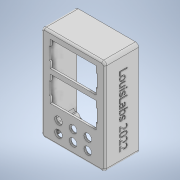
# Autodesk Inventor part: front_case
Saved by Autodesk Inventor 2022.1 (Build 261234020, 234B)
## iProperties
Created: 2022-02-06
Part Number: front_case
Material: Polylactic Acid (PLA)
Document SubType Name: Modeling
Designer: kee
Mass: 129.334 g
Surface Area: 618.34 cm^2
Volume: 103.468 cm^3
Density: 1.25 g/cm^3
Appearance: Default
Author: kee
Autodesk Inventor part; units mm, degrees
ref_plane "YZ Plane" through (0, 0, 0) normal (1, 0, 0) x (0, 1, 0)
ref_plane "XZ Plane" through (0, 0, 0) normal (0, 1, 0) x (-1, 0, 0)
ref_plane "XY Plane" through (0, 0, 0) normal (0, 0, 1) x (1, 0, 0)
sketch "Sketch1" plane through (0, 0, 0) normal (0, 0, 1) x (1, 0, 0)
  line L0 (-45, 75) -> (45, 75)
  line L1 (50, 70) -> (50, -70)
  line L2 (45, -75) -> (-45, -75)
  line L3 (-50, -70) -> (-50, 70)
  arc A0 (-45, 75) -> (-50, 70) centre (-45, 70) ccw
  arc A1 (50, 70) -> (45, 75) centre (45, 70) ccw
  arc A2 (-50, -70) -> (-45, -75) centre (-45, -70) ccw
  arc A3 (45, -75) -> (50, -70) centre (45, -70) ccw
  point P0 (0, 0)
  point P1 (-50, 75)
  point P2 (50, -75)
  point P3 (50, 75)
  point P4 (-50, -75)
  point P5 (50, 0)
  dimension "d3" = 100
  dimension "d4" = 50
  dimension "d5" = 150
  dimension "d6" = 75
  dimension "d37" = 5
  dimension "d125" = 90
  dimension "d126" = 140
  constraints: 8 end point, 8 point on circle, 8 point on line, 8 tangent, 4 centre point, 3 equal radius, 2 parallel, 1 horizontal, 1 midpoint, 1 perpendicular
  measures "d3" distance between parallel lines of L1 L3
  measures "d4" distance of point (50, 0) point (0, 0)
  measures "d5" distance between parallel lines of L2 L0
  measures "d6" distance from line of L2 point (0, 0)
  measures "d37" radius of A0
  measures "d125" distance of A0.centre A1.centre
  measures "d126" distance of A3.centre A1.centre
extrude "Extrusion1" add sketch "Sketch1" along normal blind 3
sketch "Sketch2" plane through (0, 0, 3) normal (0, 0, 1) x (1, 0, 0)
  circle A0 centre (-23, -40) radius 6
  circle A1 centre (-23, -58) radius 6
  circle A2 centre (0, -40) radius 6
  circle A3 centre (0, -58) radius 6
  circle A4 centre (23, -40) radius 6
  circle A5 centre (23, -58) radius 6
  line L0 (-45, -75) -> (45, -75) projected
  line L1 (-36, 17) -> (36, 17)
  line L2 (36, 17) -> (36, 7)
  line L3 (36, 7) -> (38, 7)
  line L4 (38, 7) -> (38, -13)
  line L5 (38, -13) -> (36, -13)
  line L6 (36, -13) -> (36, -23)
  line L7 (36, -23) -> (-36, -23)
  line L8 (-36, -23) -> (-36, -13)
  line L9 (-36, -13) -> (-38, -13)
  line L10 (-38, -13) -> (-38, 7)
  line L11 (-38, 7) -> (-36, 7)
  line L12 (-36, 17) -> (-36, 7)
  line L13 (-36, 64.5) -> (36, 64.5)
  line L14 (36, 64.5) -> (36, 54.5)
  line L15 (36, 54.5) -> (38, 54.5)
  line L16 (38, 54.5) -> (38, 34.5)
  line L17 (38, 34.5) -> (36, 34.5)
  line L18 (36, 34.5) -> (36, 24.5)
  line L19 (36, 24.5) -> (-36, 24.5)
  line L20 (-36, 24.5) -> (-36, 34.5)
  line L21 (-36, 34.5) -> (-38, 34.5)
  line L22 (-38, 34.5) -> (-38, 54.5)
  line L23 (-38, 54.5) -> (-36, 54.5)
  line L24 (-36, 64.5) -> (-36, 54.5)
  point P0 (-50, -70)
  point P1 (50, -70)
  point P2 (0, 0)
  point P3 (0, 47.5)
  dimension "d7" = 12
  dimension "d8" = 12
  dimension "d9" = 12
  dimension "d10" = 12
  dimension "d11" = 12
  dimension "d12" = 12
  dimension "d13" = 23
  dimension "d14" = 23
  dimension "d15" = 18
  dimension "d18" = 72
  dimension "d19" = 36
  dimension "d20" = 40
  dimension "d21" = 10
  dimension "d22" = 10
  dimension "d23" = 2
  dimension "d24" = 2
  dimension "d27" = 23
  dimension "d28" = 72
  dimension "d29" = 36
  dimension "d30" = 40
  dimension "d31" = 10
  dimension "d32" = 10
  dimension "d33" = 2
  dimension "d34" = 2
  dimension "d35" = 23
  dimension "d36" = 7.5
  dimension "d100" = 52
  dimension "d101" = 17
  constraints: 48 end point, 14 perpendicular, 14 point on line, 6 centre point, 4 horizontal alignment, 4 vertical alignment, 2 horizontal, 2 vertical, 1 other
  measures "d7" diameter of A0
  measures "d8" diameter of A1
  measures "d9" diameter of A2
  measures "d10" diameter of A3
  measures "d11" diameter of A4
  measures "d12" diameter of A5
  measures "d13" distance of A2.centre A0.centre
  measures "d14" distance of A4.centre A2.centre
  measures "d15" distance of A5.centre A4.centre
  measures "d18" distance of L1.start L1.end
  measures "d19" distance from line of L2 point (0, 0)
  measures "d20" distance between parallel lines of L7 L1
  measures "d21" distance of L1.end L2.end
  measures "d22" distance of L5.end L6.end
  measures "d23" distance between parallel lines of L4 L6
  measures "d24" distance between parallel lines of L10 L8
  measures "d27" distance from line of L7 point (0, 0)
  measures "d28" distance of L24.start L14.start
  measures "d29" distance from line of L14 point (0, 47.5)
  measures "d30" distance between parallel lines of L19 L13
  measures "d31" distance of L14.start L15.start
  measures "d32" distance of L18.start L19.start
  measures "d33" distance between parallel lines of L16 L18
  measures "d34" distance between parallel lines of L22 L20
  measures "d35" distance from line of L19 point (0, 47.5)
  measures "d36" distance between parallel lines of L1 L19
  measures "d100" vertical distance of point (45, -75) L6.end
  measures "d101" distance from line of L7 A4.centre
extrude "Extrusion2" cut sketch "Sketch2" against normal up to next
sketch "Sketch5" plane through (0, 0, 0) normal (0, 0, -1) x (-1, 0, 0)
  circle A0 centre (23, -40) radius 6 projected
  circle A1 centre (0, -58) radius 6 projected
  circle A2 centre (23, -58) radius 6 projected
  line L0 (38, 7) -> (38, -13) projected
  line L1 (38, -13) -> (36, -13) projected
  line L2 (36, -13) -> (36, -23) projected
  line L3 (36, -23) -> (-36, -23) projected
  line L4 (-36, -23) -> (-36, -13) projected
  line L5 (-36, -13) -> (-38, -13) projected
  line L6 (-38, -13) -> (-38, 7) projected
  line L7 (-38, 7) -> (-36, 7) projected
  line L8 (-36, 7) -> (-36, 17) projected
  line L9 (-36, 17) -> (36, 17) projected
  line L10 (36, 17) -> (36, 7) projected
  line L11 (36, 7) -> (38, 7) projected
  circle A3 centre (0, -40) radius 6 projected
  circle A4 centre (-23, -58) radius 6 projected
  circle A5 centre (-23, -40) radius 6 projected
  line L12 (38, 54.5) -> (38, 34.5) projected
  line L13 (38, 34.5) -> (36, 34.5) projected
  line L14 (36, 34.5) -> (36, 24.5) projected
  line L15 (36, 24.5) -> (-36, 24.5) projected
  line L16 (-36, 24.5) -> (-36, 34.5) projected
  line L17 (-36, 34.5) -> (-38, 34.5) projected
  line L18 (-38, 34.5) -> (-38, 54.5) projected
  line L19 (-38, 54.5) -> (-36, 54.5) projected
  line L20 (-36, 54.5) -> (-36, 64.5) projected
  line L21 (-36, 64.5) -> (36, 64.5) projected
  line L22 (36, 64.5) -> (36, 54.5) projected
  line L23 (36, 54.5) -> (38, 54.5) projected
  line L24 (45, -75) -> (-45, -75) projected
  arc A6 (45, -75) -> (50, -70) centre (45, -70) ccw projected
  line L25 (50, 70) -> (50, -70) projected
  arc A7 (50, 70) -> (45, 75) centre (45, 70) ccw projected
  line L26 (-45, 75) -> (45, 75) projected
  arc A8 (-45, 75) -> (-50, 70) centre (-45, 70) ccw projected
  line L27 (-50, -70) -> (-50, 70) projected
  arc A9 (-50, -70) -> (-45, -75) centre (-45, -70) ccw projected
  arc A10 (47, 70) -> (45, 72) centre (45, 70) ccw
  line L28 (47, 70) -> (47, -70)
  arc A11 (45, -72) -> (47, -70) centre (45, -70) ccw
  line L29 (45, -72) -> (-45, -72)
  arc A12 (-47, -70) -> (-45, -72) centre (-45, -70) ccw
  line L30 (-47, -70) -> (-47, 70)
  arc A13 (-45, 72) -> (-47, 70) centre (-45, 70) ccw
  line L31 (-45, 72) -> (45, 72)
  line L32 (-45, 75) -> (45, 75)
  arc A14 (50, 70) -> (45, 75) centre (45, 70) ccw
  line L33 (50, 70) -> (50, -70)
  arc A15 (45, -75) -> (50, -70) centre (45, -70) ccw
  line L34 (45, -75) -> (-45, -75)
  arc A16 (-50, -70) -> (-45, -75) centre (-45, -70) ccw
  line L35 (-50, -70) -> (-50, 70)
  arc A17 (-45, 75) -> (-50, 70) centre (-45, 70) ccw
  line L36 (-116.3396, 0) -> (109.1655, 0) construction
  line L37 (0, 86.6309) -> (0, -88.1774) construction
  line L38 (-47, 62) -> (-42, 62)
  line L39 (-37, 67) -> (-37, 72)
  arc A18 (-42, 62) -> (-37, 67) centre (-42, 67) ccw
  line L40 (47, 62) -> (42, 62)
  line L41 (37, 67) -> (37, 72)
  arc A19 (37, 67) -> (42, 62) centre (42, 67) ccw
  line L42 (37, -72) -> (37, -67)
  line L43 (42, -62) -> (47, -62)
  arc A20 (42, -62) -> (37, -67) centre (42, -67) ccw
  line L44 (-37, -72) -> (-37, -67)
  line L45 (-42, -62) -> (-47, -62)
  arc A21 (-37, -67) -> (-42, -62) centre (-42, -67) ccw
  point P0 (0, 0)
  point P1 (-37, 62)
  point P2 (37, 62)
  point P3 (37, -62)
  point P4 (-37, -62)
  dimension "d38" = 3
  dimension "d103" = 10
  dimension "d104" = 10
  dimension "d105" = 5
  dimension "d108" = 10
  dimension "d109" = 10
  dimension "d110" = 5
  dimension "d111" = 10
  dimension "d112" = 10
  dimension "d113" = 5
  dimension "d114" = 10
  dimension "d115" = 10
  dimension "d116" = 5
  dimension "d127" = 84
  dimension "d128" = 134
  constraints: 36 end point, 24 point on circle, 18 point on line, 13 tangent, 12 centre point, 5 perpendicular, 4 coincident, 4 horizontal, 4 vertical, 7 other
  measures "d38" distance between parallel lines of L26 L31
  measures "d103" distance of L38.start point (-37, 62)
  measures "d104" distance of point (-37, 62) L39.end
  measures "d105" radius of A18
  measures "d108" distance of L40.start point (37, 62)
  measures "d109" distance of point (37, 62) L41.end
  measures "d110" radius of A19
  measures "d111" distance of L42.start point (37, -62)
  measures "d112" distance of point (37, -62) L43.end
  measures "d113" radius of A20
  measures "d114" distance of L44.start point (-37, -62)
  measures "d115" distance of point (-37, -62) L45.end
  measures "d116" radius of A21
  measures "d127" distance of A19.centre A18.centre
  measures "d128" distance of A20.centre A19.centre
extrude "Extrusion13" add sketch "Sketch5" along normal blind 50 contours L24 A9 L27 A8 L26 A7 L25 A6 | L28 L40 A19 L41 L31 A10 | L28 A11 L29 L42 A20 L43 | L39 A18 L38 L30 A13 L31 | L29 A12 L30 L45 A21 L44
sketch "Sketch17" plane through (0, 0, -50) normal (0, 0, -1) x (-1, 0, 0)
  line L0 (-45, -75) -> (45, -75) projected
  arc A0 (45, -75) -> (50, -70) centre (45, -70) ccw projected
  line L1 (50, -70) -> (50, 70) projected
  arc A1 (50, 70) -> (45, 75) centre (45, 70) ccw projected
  line L2 (45, 75) -> (-45, 75) projected
  arc A2 (-45, 75) -> (-50, 70) centre (-45, 70) ccw projected
  line L3 (-50, 70) -> (-50, -70) projected
  arc A3 (-50, -70) -> (-45, -75) centre (-45, -70) ccw projected
  line L4 (37, 72) -> (37, 67) projected
  arc A4 (37, 67) -> (42, 62) centre (42, 67) ccw projected
  line L5 (42, 62) -> (47, 62) projected
  line L6 (47, 62) -> (47, -62) projected
  line L7 (47, -62) -> (42, -62) projected
  arc A5 (42, -62) -> (37, -67) centre (42, -67) ccw projected
  line L8 (37, -67) -> (37, -72) projected
  line L9 (37, -72) -> (-37, -72) projected
  line L10 (-37, -72) -> (-37, -67) projected
  arc A6 (-37, -67) -> (-42, -62) centre (-42, -67) ccw projected
  line L11 (-42, -62) -> (-47, -62) projected
  line L12 (-47, -62) -> (-47, 62) projected
  line L13 (-47, 62) -> (-42, 62) projected
  arc A7 (-42, 62) -> (-37, 67) centre (-42, 67) ccw projected
  line L14 (-37, 67) -> (-37, 72) projected
  line L15 (-37, 72) -> (37, 72) projected
  line L16 (-42, 72) -> (42, 72)
  line L17 (47, 67) -> (47, -67)
  line L18 (42, -72) -> (-42, -72)
  line L19 (-47, -67) -> (-47, 67)
  arc A8 (-42, 72) -> (-47, 67) centre (-42, 67) ccw
  arc A9 (47, 67) -> (42, 72) centre (42, 67) ccw
  arc A10 (42, -72) -> (47, -67) centre (42, -67) ccw
  arc A11 (-47, -67) -> (-42, -72) centre (-42, -67) ccw
  point P0 (0, 0)
  point P1 (-47, 72)
  point P2 (-47, 62)
  dimension "d117" = 5
  constraints: 8 end point, 8 point on circle, 8 tangent, 4 centre point, 3 equal radius, 3 point on line, 2 parallel, 1 horizontal, 1 perpendicular
  measures "d117" radius of A8
extrude "Extrusion14" cut sketch "Sketch17" against normal blind 5 contours L16 A9 L17 L5 A4 L4 | L4 A4 L5 L6 L7 A5 L8 L9 L10 A6 L11 L12 L13 A7 L14 L15 | L14 A7 L13 L19 A8 L16 | L17 A10 L18 L8 A5 L7 | L11 A6 L10 L18 A11 L19
sketch "Sketch18" plane through (-45, -75, 3) normal (0, -1, 0) x (1, 0, 0)
  line L0 (3, -53) -> (87, -53) projected
  line L1 (85, -53) -> (5, -53)
  line L2 (5, -53) -> (5, -10)
  line L3 (5, -10) -> (85, -10)
  line L4 (85, -10) -> (85, -53)
  line L5 (0, 0) -> (90, 0) projected
  line L6 (45, -65.8831) -> (45, 5.9535) construction
  point P0 (45, -3)
  point P1 (45, 0)
  point P2 (5, -53)
  dimension "d120" = 10
  dimension "d121" = 80
  dimension "d122" = 40
  constraints: 10 end point, 2 parallel, 2 point on line, 1 horizontal, 1 midpoint, 1 perpendicular, 1 vertical
  measures "d120" distance between parallel lines of L5 L3
  measures "d121" distance between parallel lines of L2 L4
  measures "d122" distance between parallel lines of L2 L6
extrude "Extrusion15" cut sketch "Sketch18" against normal up to surface (3 mm away)
fillet "Fillet1" radius 3 2 edges at (40, -73.5, -7) (-40, -73.5, -7)
sketch "Sketch19" plane through (0, 0, -45) normal (0, 0, -1) x (-1, 0, 0)
  line L0 (-42, 62) -> (-47, 62) construction
  arc A0 (-42, 62) -> (-37, 67) centre (-42, 67) ccw construction
  line L1 (-37, 72) -> (-37, 67) construction
  line L2 (-42, 72) -> (-37, 72) construction
  arc A1 (-42, 72) -> (-47, 67) centre (-42, 67) ccw construction
  line L3 (-47, 62) -> (-47, 67) construction
  line L4 (47, 62) -> (42, 62) construction
  line L5 (47, 67) -> (47, 62) construction
  arc A2 (47, 67) -> (42, 72) centre (42, 67) ccw construction
  line L6 (37, 72) -> (42, 72) construction
  line L7 (37, 67) -> (37, 72) construction
  arc A3 (37, 67) -> (42, 62) centre (42, 67) ccw construction
  line L8 (37, -72) -> (37, -67) construction
  line L9 (40, -72) -> (37, -72) construction
  line L10 (42, -72) -> (40, -72) construction
  arc A4 (42, -72) -> (47, -67) centre (42, -67) ccw construction
  line L11 (47, -62) -> (47, -67) construction
  line L12 (42, -62) -> (47, -62) construction
  arc A5 (42, -62) -> (37, -67) centre (42, -67) ccw construction
  line L13 (-37, -67) -> (-37, -72) construction
  arc A6 (-37, -67) -> (-42, -62) centre (-42, -67) ccw construction
  line L14 (-47, -62) -> (-42, -62) construction
  line L15 (-47, -67) -> (-47, -62) construction
  arc A7 (-47, -67) -> (-42, -72) centre (-42, -67) ccw construction
  line L16 (-40, -72) -> (-42, -72) construction
  line L17 (-37, -72) -> (-40, -72) construction
  point P0 (0, 0)
hole "Hole1" at (42, 67, -45) at (-42, 67, -45) at (-42, -67, -45) at (42, -67, -45) direction (0, 0, 1) diameter 3 depth 15 tip angle 118
fillet "Fillet2" radius 3 29 edges at (48.5355, 73.5355, 3) (0, 75, 3) (-48.5355, 73.5355, 3) (-50, 0, 3) (-48.5355, -73.5355, 3) (0, -75, 3) (48.5355, -73.5355, 3) (50, 0, 3) (47, 62, -22.5) (37, 72, -22.5) (-47, 62, -22.5) (-37, 72, -22.5) (-47, -62, -22.5) (47, -62, -22.5) (47, 0, 0) (37, -69.5, 0) (44.5, -62, 0) (38.4645, -63.4645, 0) (-38.4645, -63.4645, 0) (-44.5, -62, 0) (-37, -69.5, 0) (0, -72, 0) (0, 72, 0) (38.4645, 63.4645, 0) (44.5, 62, 0) (37, 69.5, 0) (-38.4645, 63.4645, 0) (-44.5, 62, 0) (-37, 69.5, 0)
sketch "Sketch20" plane through (50, -70, -50) normal (1, 0, 0) x (0, 0, -1)
  line L0 (-30.2308, 115.0433) -> (-30.2308, 121.9963)
  line L1 (-30.2308, 121.9963) -> (-18.2308, 121.9963)
  line L2 (-18.2308, 121.9963) -> (-18.2308, 120.4015)
  line L3 (-18.2308, 120.4015) -> (-28.811, 120.4015)
  line L4 (-28.811, 120.4015) -> (-28.811, 115.0433)
  line L5 (-28.811, 115.0433) -> (-30.2308, 115.0433)
  spline S0 degree 2 poles (-25.7284, 106.5052) (-28.0039, 106.5052) (-30.4836, 108.6932) (-30.4836, 110.5214) knots 0 0 0 1 2 2 2
  spline S1 degree 2 poles (-30.4836, 110.5214) (-30.4836, 112.3982) (-27.9261, 114.5474) (-25.7284, 114.5474) knots 0 0 0 1 2 2 2
  spline S2 degree 2 poles (-25.7284, 114.5474) (-23.4723, 114.5474) (-20.9731, 112.3302) (-20.9731, 110.5214) knots 0 0 0 1 2 2 2
  spline S3 degree 2 poles (-20.9731, 110.5214) (-20.9731, 108.6932) (-23.4626, 106.5052) (-25.7284, 106.5052) knots 0 0 0 1 2 2 2
  spline S4 degree 2 poles (-25.7284, 108.0709) (-23.9779, 108.0709) (-22.2762, 109.3448) (-22.2762, 110.5214) knots 0 0 0 1 2 2 2
  spline S5 degree 2 poles (-22.2762, 110.5214) (-22.2762, 111.6981) (-23.9779, 112.9817) (-25.7284, 112.9817) knots 0 0 0 1 2 2 2
  spline S6 degree 2 poles (-25.7284, 112.9817) (-27.4301, 112.9817) (-29.1805, 111.6981) (-29.1805, 110.5214) knots 0 0 0 1 2 2 2
  spline S7 degree 2 poles (-29.1805, 110.5214) (-29.1805, 109.3545) (-27.4593, 108.0709) (-25.7284, 108.0709) knots 0 0 0 1 2 2 2
  line L6 (-30.2308, 97.9477) -> (-30.2308, 99.4647)
  line L7 (-30.2308, 99.4647) -> (-29.2389, 99.4647)
  spline S8 degree 2 poles (-29.2389, 99.4647) (-29.8515, 100.1649) (-30.4836, 101.4193) (-30.4836, 102.1973) knots 0 0 0 1 2 2 2
  spline S9 degree 2 poles (-30.4836, 102.1973) (-30.4836, 102.7807) (-30.0946, 103.8213) (-29.6765, 104.2005) knots 0 0 0 1 2 2 2
  spline S10 degree 2 poles (-29.6765, 104.2005) (-29.2583, 104.5895) (-27.9844, 105.0174) (-27.0703, 105.0174) knots 0 0 0 1 2 2 2
  line L8 (-27.0703, 105.0174) -> (-21.2259, 105.0174)
  line L9 (-21.2259, 105.0174) -> (-21.2259, 103.5004)
  line L10 (-21.2259, 103.5004) -> (-26.3604, 103.5004)
  spline S11 degree 2 poles (-26.3604, 103.5004) (-27.0801, 103.5004) (-28.0233, 103.3934) (-28.3734, 103.2086) knots 0 0 0 1 2 2 2
  spline S12 degree 2 poles (-28.3734, 103.2086) (-28.7235, 103.0239) (-29.0444, 102.3918) (-29.0444, 101.7986) knots 0 0 0 1 2 2 2
  spline S13 degree 2 poles (-29.0444, 101.7986) (-29.0444, 101.2443) (-28.4123, 99.9898) (-27.9553, 99.4647) knots 0 0 0 1 2 2 2
  line L11 (-27.9553, 99.4647) -> (-21.2259, 99.4647)
  line L12 (-21.2259, 99.4647) -> (-21.2259, 97.9477)
  line L13 (-21.2259, 97.9477) -> (-30.2308, 97.9477)
  line L14 (-30.2308, 94.2038) -> (-30.2308, 95.7208)
  line L15 (-30.2308, 95.7208) -> (-21.2259, 95.7208)
  line L16 (-21.2259, 95.7208) -> (-21.2259, 94.2038)
  line L17 (-21.2259, 94.2038) -> (-30.2308, 94.2038)
  line L18 (-19.7284, 94.0968) -> (-19.7284, 95.818)
  line L19 (-19.7284, 95.818) -> (-18.153, 95.818)
  line L20 (-18.153, 95.818) -> (-18.153, 94.0968)
  line L21 (-18.153, 94.0968) -> (-19.7284, 94.0968)
  spline S14 degree 2 poles (-30.4447, 89.5457) (-30.4447, 90.4501) (-29.9585, 92.0158) (-29.6862, 92.5311) knots 0 0 0 1 2 2 2
  line L22 (-29.6862, 92.5311) -> (-27.9844, 92.5311)
  line L23 (-27.9844, 92.5311) -> (-27.9844, 92.4534)
  spline S15 degree 2 poles (-27.9844, 92.4534) (-28.14, 92.2589) (-28.5096, 91.7337) (-28.7138, 91.2961) knots 0 0 0 1 2 2 2
  spline S16 degree 2 poles (-28.7138, 91.2961) (-28.8985, 90.9169) (-29.1708, 89.9833) (-29.1708, 89.4874) knots 0 0 0 1 2 2 2
  spline S17 degree 2 poles (-29.1708, 89.4874) (-29.1708, 89.1276) (-29.0055, 88.301) (-28.8694, 88.1065) knots 0 0 0 1 2 2 2
  spline S18 degree 2 poles (-28.8694, 88.1065) (-28.6846, 87.8245) (-28.2664, 87.5717) (-27.8386, 87.5717) knots 0 0 0 1 2 2 2
  spline S19 degree 2 poles (-27.8386, 87.5717) (-27.3037, 87.5717) (-26.7494, 88.1551) (-26.5647, 88.9039) knots 0 0 0 1 2 2 2
  spline S20 degree 2 poles (-26.5647, 88.9039) (-26.4966, 89.1957) (-26.3021, 90.1292) (-26.1951, 90.5279) knots 0 0 0 1 2 2 2
  spline S21 degree 2 poles (-26.1951, 90.5279) (-25.8937, 91.5587) (-24.6489, 92.4923) (-23.764, 92.4923) knots 0 0 0 1 2 2 2
  spline S22 degree 2 poles (-23.764, 92.4923) (-22.5387, 92.4923) (-21.012, 90.6543) (-21.012, 89.1373) knots 0 0 0 1 2 2 2
  spline S23 degree 2 poles (-21.012, 89.1373) (-21.012, 88.3885) (-21.3815, 86.8715) (-21.6635, 86.3561) knots 0 0 0 1 2 2 2
  line L24 (-21.6635, 86.3561) -> (-23.2875, 86.3561)
  line L25 (-23.2875, 86.3561) -> (-23.2875, 86.4339)
  spline S24 degree 2 poles (-23.2875, 86.4339) (-22.8207, 87.0174) (-22.2859, 88.4371) (-22.2859, 89.1665) knots 0 0 0 1 2 2 2
  spline S25 degree 2 poles (-22.2859, 89.1665) (-22.2859, 89.9153) (-22.918, 90.9461) (-23.5501, 90.9461) knots 0 0 0 1 2 2 2
  spline S26 degree 2 poles (-23.5501, 90.9461) (-24.1238, 90.9461) (-24.6781, 90.3334) (-24.8532, 89.6527) knots 0 0 0 1 2 2 2
  spline S27 degree 2 poles (-24.8532, 89.6527) (-24.9407, 89.3221) (-25.1157, 88.4858) (-25.2227, 88.0287) knots 0 0 0 1 2 2 2
  spline S28 degree 2 poles (-25.2227, 88.0287) (-25.4755, 87.0368) (-26.6327, 86.0255) (-27.6343, 86.0255) knots 0 0 0 1 2 2 2
  spline S29 degree 2 poles (-27.6343, 86.0255) (-28.2178, 86.0255) (-29.2486, 86.4825) (-29.6279, 86.9299) knots 0 0 0 1 2 2 2
  spline S30 degree 2 poles (-29.6279, 86.9299) (-30.0266, 87.4064) (-30.4447, 88.6219) (-30.4447, 89.5457) knots 0 0 0 1 2 2 2
  line L26 (-30.2308, 77.5457) -> (-30.2308, 84.4987)
  line L27 (-30.2308, 84.4987) -> (-18.2308, 84.4987)
  line L28 (-18.2308, 84.4987) -> (-18.2308, 82.9039)
  line L29 (-18.2308, 82.9039) -> (-28.811, 82.9039)
  line L30 (-28.811, 82.9039) -> (-28.811, 77.5457)
  line L31 (-28.811, 77.5457) -> (-30.2308, 77.5457)
  spline S31 degree 2 poles (-29.2778, 71.3901) (-29.4139, 71.5749) (-29.9002, 72.1973) (-30.046, 72.489) knots 0 0 0 1 2 2 2
  spline S32 degree 2 poles (-30.046, 72.489) (-30.26, 72.8877) (-30.4836, 73.6365) (-30.4836, 74.3172) knots 0 0 0 1 2 2 2
  spline S33 degree 2 poles (-30.4836, 74.3172) (-30.4836, 74.8715) (-30.0655, 75.8731) (-29.6862, 76.2524) knots 0 0 0 1 2 2 2
  spline S34 degree 2 poles (-29.6862, 76.2524) (-29.3167, 76.6122) (-28.2275, 77.0498) (-27.6246, 77.0498) knots 0 0 0 1 2 2 2
  spline S35 degree 2 poles (-27.6246, 77.0498) (-26.6911, 77.0498) (-25.3685, 76.2621) (-24.9893, 75.4064) knots 0 0 0 1 2 2 2
  spline S36 degree 2 poles (-24.9893, 75.4064) (-24.6392, 74.6478) (-24.3767, 72.5863) (-24.3086, 71.3901) knots 0 0 0 1 2 2 2
  line L32 (-24.3086, 71.3901) -> (-24.0168, 71.3901)
  spline S37 degree 2 poles (-24.0168, 71.3901) (-23.4917, 71.3901) (-22.8402, 71.7111) (-22.6554, 72.0028) knots 0 0 0 1 2 2 2
  spline S38 degree 2 poles (-22.6554, 72.0028) (-22.4707, 72.2945) (-22.354, 73.1308) (-22.354, 73.5782) knots 0 0 0 1 2 2 2
  spline S39 degree 2 poles (-22.354, 73.5782) (-22.354, 74.1033) (-22.6651, 75.523) (-22.9666, 76.2329) knots 0 0 0 1 2 2 2
  line L33 (-22.9666, 76.2329) -> (-22.9666, 76.3205)
  line L34 (-22.9666, 76.3205) -> (-21.4204, 76.3205)
  spline S40 degree 2 poles (-21.4204, 76.3205) (-21.3037, 75.9023) (-21.012, 74.3367) (-21.012, 73.5684) knots 0 0 0 1 2 2 2
  spline S41 degree 2 poles (-21.012, 73.5684) (-21.012, 72.6349) (-21.3037, 71.361) (-21.683, 70.8553) knots 0 0 0 1 2 2 2
  spline S42 degree 2 poles (-21.683, 70.8553) (-22.0525, 70.3593) (-23.2292, 69.8731) (-24.0752, 69.8731) knots 0 0 0 1 2 2 2
  line L35 (-24.0752, 69.8731) -> (-30.2308, 69.8731)
  line L36 (-30.2308, 69.8731) -> (-30.2308, 71.3901)
  line L37 (-30.2308, 71.3901) -> (-29.2778, 71.3901)
  line L38 (-28.0136, 71.3901) -> (-25.5144, 71.3901)
  spline S43 degree 2 poles (-25.5144, 71.3901) (-25.563, 71.9347) (-25.7284, 73.5782) (-25.8839, 74.0935) knots 0 0 0 1 2 2 2
  spline S44 degree 2 poles (-25.8839, 74.0935) (-26.0687, 74.6965) (-26.8369, 75.4841) (-27.5177, 75.4841) knots 0 0 0 1 2 2 2
  spline S45 degree 2 poles (-27.5177, 75.4841) (-28.2956, 75.4841) (-29.0833, 74.6089) (-29.0833, 73.7726) knots 0 0 0 1 2 2 2
  spline S46 degree 2 poles (-29.0833, 73.7726) (-29.0833, 73.0628) (-28.4707, 71.8958) (-28.0136, 71.3901) knots 0 0 0 1 2 2 2
  spline S47 degree 2 poles (-25.5825, 60.1973) (-27.7899, 60.1973) (-30.4836, 62.3367) (-30.4836, 63.9509) knots 0 0 0 1 2 2 2
  spline S48 degree 2 poles (-30.4836, 63.9509) (-30.4836, 64.6803) (-30.1238, 65.7208) (-29.8126, 66.2264) knots 0 0 0 1 2 2 2
  line L39 (-29.8126, 66.2264) -> (-30.2308, 66.3237)
  line L40 (-30.2308, 66.3237) -> (-30.2308, 67.7435)
  line L41 (-30.2308, 67.7435) -> (-17.6959, 67.7435)
  line L42 (-17.6959, 67.7435) -> (-17.6959, 66.2264)
  line L43 (-17.6959, 66.2264) -> (-22.1692, 66.2264)
  spline S49 degree 2 poles (-22.1692, 66.2264) (-21.6538, 65.6527) (-20.9731, 64.3205) (-20.9731, 63.4744) knots 0 0 0 1 2 2 2
  spline S50 degree 2 poles (-20.9731, 63.4744) (-20.9731, 61.9477) (-23.4139, 60.1973) (-25.5825, 60.1973) knots 0 0 0 1 2 2 2
  spline S51 degree 2 poles (-25.6992, 61.7629) (-24.0849, 61.7629) (-22.4123, 62.7451) (-22.4123, 63.8342) knots 0 0 0 1 2 2 2
  spline S52 degree 2 poles (-22.4123, 63.8342) (-22.4123, 64.4469) (-22.9958, 65.7111) (-23.4431, 66.2264) knots 0 0 0 1 2 2 2
  line L44 (-23.4431, 66.2264) -> (-28.6068, 66.2264)
  spline S53 degree 2 poles (-28.6068, 66.2264) (-28.8888, 65.6527) (-29.1222, 64.7678) (-29.1222, 64.2427) knots 0 0 0 1 2 2 2
  spline S54 degree 2 poles (-29.1222, 64.2427) (-29.1222, 63.0854) (-27.4788, 61.7629) (-25.6992, 61.7629) knots 0 0 0 1 2 2 2
  spline S55 degree 2 poles (-30.4447, 56.1908) (-30.4447, 57.0952) (-29.9585, 58.6608) (-29.6862, 59.1762) knots 0 0 0 1 2 2 2
  line L45 (-29.6862, 59.1762) -> (-27.9844, 59.1762)
  line L46 (-27.9844, 59.1762) -> (-27.9844, 59.0984)
  spline S56 degree 2 poles (-27.9844, 59.0984) (-28.14, 58.9039) (-28.5096, 58.3788) (-28.7138, 57.9412) knots 0 0 0 1 2 2 2
  spline S57 degree 2 poles (-28.7138, 57.9412) (-28.8985, 57.5619) (-29.1708, 56.6284) (-29.1708, 56.1324) knots 0 0 0 1 2 2 2
  spline S58 degree 2 poles (-29.1708, 56.1324) (-29.1708, 55.7726) (-29.0055, 54.9461) (-28.8694, 54.7516) knots 0 0 0 1 2 2 2
  spline S59 degree 2 poles (-28.8694, 54.7516) (-28.6846, 54.4696) (-28.2664, 54.2167) (-27.8386, 54.2167) knots 0 0 0 1 2 2 2
  spline S60 degree 2 poles (-27.8386, 54.2167) (-27.3037, 54.2167) (-26.7494, 54.8002) (-26.5647, 55.549) knots 0 0 0 1 2 2 2
  spline S61 degree 2 poles (-26.5647, 55.549) (-26.4966, 55.8407) (-26.3021, 56.7743) (-26.1951, 57.173) knots 0 0 0 1 2 2 2
  spline S62 degree 2 poles (-26.1951, 57.173) (-25.8937, 58.2038) (-24.6489, 59.1373) (-23.764, 59.1373) knots 0 0 0 1 2 2 2
  spline S63 degree 2 poles (-23.764, 59.1373) (-22.5387, 59.1373) (-21.012, 57.2994) (-21.012, 55.7824) knots 0 0 0 1 2 2 2
  spline S64 degree 2 poles (-21.012, 55.7824) (-21.012, 55.0336) (-21.3815, 53.5166) (-21.6635, 53.0012) knots 0 0 0 1 2 2 2
  line L47 (-21.6635, 53.0012) -> (-23.2875, 53.0012)
  line L48 (-23.2875, 53.0012) -> (-23.2875, 53.079)
  spline S65 degree 2 poles (-23.2875, 53.079) (-22.8207, 53.6624) (-22.2859, 55.0822) (-22.2859, 55.8115) knots 0 0 0 1 2 2 2
  spline S66 degree 2 poles (-22.2859, 55.8115) (-22.2859, 56.5603) (-22.918, 57.5911) (-23.5501, 57.5911) knots 0 0 0 1 2 2 2
  spline S67 degree 2 poles (-23.5501, 57.5911) (-24.1238, 57.5911) (-24.6781, 56.9785) (-24.8532, 56.2978) knots 0 0 0 1 2 2 2
  spline S68 degree 2 poles (-24.8532, 56.2978) (-24.9407, 55.9671) (-25.1157, 55.1308) (-25.2227, 54.6738) knots 0 0 0 1 2 2 2
  spline S69 degree 2 poles (-25.2227, 54.6738) (-25.4755, 53.6819) (-26.6327, 52.6705) (-27.6343, 52.6705) knots 0 0 0 1 2 2 2
  spline S70 degree 2 poles (-27.6343, 52.6705) (-28.2178, 52.6705) (-29.2486, 53.1276) (-29.6279, 53.5749) knots 0 0 0 1 2 2 2
  spline S71 degree 2 poles (-29.6279, 53.5749) (-30.0266, 54.0514) (-30.4447, 55.267) (-30.4447, 56.1908) knots 0 0 0 1 2 2 2
  line L49 (-30.2308, 38.9299) -> (-30.2308, 46.3302)
  line L50 (-30.2308, 46.3302) -> (-28.529, 46.3302)
  spline S72 degree 2 poles (-28.529, 46.3302) (-27.7802, 45.5328) (-26.3896, 44.113) (-25.6408, 43.4323) knots 0 0 0 1 2 2 2
  spline S73 degree 2 poles (-25.6408, 43.4323) (-24.1335, 42.0611) (-22.3248, 41.0595) (-21.3621, 41.0595) knots 0 0 0 1 2 2 2
  spline S74 degree 2 poles (-21.3621, 41.0595) (-20.8564, 41.0595) (-20.0979, 41.3707) (-19.8548, 41.6527) knots 0 0 0 1 2 2 2
  spline S75 degree 2 poles (-19.8548, 41.6527) (-19.6117, 41.9347) (-19.3685, 42.6738) (-19.3685, 43.1211) knots 0 0 0 1 2 2 2
  spline S76 degree 2 poles (-19.3685, 43.1211) (-19.3685, 43.549) (-19.5825, 44.4242) (-19.7478, 44.8229) knots 0 0 0 1 2 2 2
  spline S77 degree 2 poles (-19.7478, 44.8229) (-19.8839, 45.1632) (-20.2729, 45.7953) (-20.4091, 45.9898) knots 0 0 0 1 2 2 2
  line L51 (-20.4091, 45.9898) -> (-20.4091, 46.0773)
  line L52 (-20.4091, 46.0773) -> (-18.6976, 46.0773)
  spline S78 degree 2 poles (-18.6976, 46.0773) (-18.4544, 45.5814) (-17.9779, 43.8018) (-17.9779, 43.0044) knots 0 0 0 1 2 2 2
  spline S79 degree 2 poles (-17.9779, 43.0044) (-17.9779, 41.3221) (-19.7575, 39.4258) (-21.2745, 39.4258) knots 0 0 0 1 2 2 2
  spline S80 degree 2 poles (-21.2745, 39.4258) (-21.9844, 39.4258) (-23.1708, 39.7564) (-23.6765, 40.0482) knots 0 0 0 1 2 2 2
  spline S81 degree 2 poles (-23.6765, 40.0482) (-24.2016, 40.3399) (-25.2324, 41.1859) (-25.7284, 41.6527) knots 0 0 0 1 2 2 2
  spline S82 degree 2 poles (-25.7284, 41.6527) (-26.5549, 42.4112) (-28.3248, 44.2686) (-28.8402, 44.8229) knots 0 0 0 1 2 2 2
  line L53 (-28.8402, 44.8229) -> (-28.8402, 38.9299)
  line L54 (-28.8402, 38.9299) -> (-30.2308, 38.9299)
  spline S83 degree 2 poles (-24.2308, 29.8569) (-27.4593, 29.8569) (-30.4836, 31.7337) (-30.4836, 33.6884) knots 0 0 0 1 2 2 2
  spline S84 degree 2 poles (-30.4836, 33.6884) (-30.4836, 35.6722) (-27.401, 37.5295) (-24.2405, 37.5295) knots 0 0 0 1 2 2 2
  spline S85 degree 2 poles (-24.2405, 37.5295) (-20.9925, 37.5295) (-17.9877, 35.6527) (-17.9877, 33.6884) knots 0 0 0 1 2 2 2
  spline S86 degree 2 poles (-17.9877, 33.6884) (-17.9877, 31.7143) (-21.0995, 29.8569) (-24.2308, 29.8569) knots 0 0 0 1 2 2 2
  spline S87 degree 2 poles (-27.8872, 31.9185) (-27.294, 31.6851) (-25.4658, 31.4906) (-24.2308, 31.4906) knots 0 0 0 1 2 2 2
  spline S88 degree 2 poles (-24.2308, 31.4906) (-22.9958, 31.4906) (-21.1773, 31.6851) (-20.5647, 31.9282) knots 0 0 0 1 2 2 2
  spline S89 degree 2 poles (-20.5647, 31.9282) (-19.952, 32.1713) (-19.3199, 33.0174) (-19.3199, 33.6884) knots 0 0 0 1 2 2 2
  spline S90 degree 2 poles (-19.3199, 33.6884) (-19.3199, 34.3593) (-19.952, 35.2248) (-20.5841, 35.4777) knots 0 0 0 1 2 2 2
  spline S91 degree 2 poles (-20.5841, 35.4777) (-21.1967, 35.7208) (-23.0638, 35.8958) (-24.2405, 35.8958) knots 0 0 0 1 2 2 2
  spline S92 degree 2 poles (-24.2405, 35.8958) (-25.5047, 35.8958) (-27.1967, 35.7402) (-27.858, 35.4874) knots 0 0 0 1 2 2 2
  spline S93 degree 2 poles (-27.858, 35.4874) (-28.4804, 35.254) (-29.1514, 34.3885) (-29.1514, 33.6884) knots 0 0 0 1 2 2 2
  spline S94 degree 2 poles (-29.1514, 33.6884) (-29.1514, 33.0271) (-28.5193, 32.1616) (-27.8872, 31.9185) knots 0 0 0 1 2 2 2
  line L55 (-30.2308, 20.9201) -> (-30.2308, 28.3205)
  line L56 (-30.2308, 28.3205) -> (-28.529, 28.3205)
  spline S95 degree 2 poles (-28.529, 28.3205) (-27.7802, 27.523) (-26.3896, 26.1033) (-25.6408, 25.4226) knots 0 0 0 1 2 2 2
  spline S96 degree 2 poles (-25.6408, 25.4226) (-24.1335, 24.0514) (-22.3248, 23.0498) (-21.3621, 23.0498) knots 0 0 0 1 2 2 2
  spline S97 degree 2 poles (-21.3621, 23.0498) (-20.8564, 23.0498) (-20.0979, 23.361) (-19.8548, 23.643) knots 0 0 0 1 2 2 2
  spline S98 degree 2 poles (-19.8548, 23.643) (-19.6117, 23.925) (-19.3685, 24.664) (-19.3685, 25.1114) knots 0 0 0 1 2 2 2
  spline S99 degree 2 poles (-19.3685, 25.1114) (-19.3685, 25.5393) (-19.5825, 26.4145) (-19.7478, 26.8132) knots 0 0 0 1 2 2 2
  spline S100 degree 2 poles (-19.7478, 26.8132) (-19.8839, 27.1535) (-20.2729, 27.7856) (-20.4091, 27.9801) knots 0 0 0 1 2 2 2
  line L57 (-20.4091, 27.9801) -> (-20.4091, 28.0676)
  line L58 (-20.4091, 28.0676) -> (-18.6976, 28.0676)
  spline S101 degree 2 poles (-18.6976, 28.0676) (-18.4544, 27.5717) (-17.9779, 25.7921) (-17.9779, 24.9947) knots 0 0 0 1 2 2 2
  spline S102 degree 2 poles (-17.9779, 24.9947) (-17.9779, 23.3123) (-19.7575, 21.4161) (-21.2745, 21.4161) knots 0 0 0 1 2 2 2
  spline S103 degree 2 poles (-21.2745, 21.4161) (-21.9844, 21.4161) (-23.1708, 21.7467) (-23.6765, 22.0384) knots 0 0 0 1 2 2 2
  spline S104 degree 2 poles (-23.6765, 22.0384) (-24.2016, 22.3302) (-25.2324, 23.1762) (-25.7284, 23.643) knots 0 0 0 1 2 2 2
  spline S105 degree 2 poles (-25.7284, 23.643) (-26.5549, 24.4015) (-28.3248, 26.2589) (-28.8402, 26.8132) knots 0 0 0 1 2 2 2
  line L59 (-28.8402, 26.8132) -> (-28.8402, 20.9201)
  line L60 (-28.8402, 20.9201) -> (-30.2308, 20.9201)
  line L61 (-30.2308, 11.9153) -> (-30.2308, 19.3156)
  line L62 (-30.2308, 19.3156) -> (-28.529, 19.3156)
  spline S106 degree 2 poles (-28.529, 19.3156) (-27.7802, 18.5182) (-26.3896, 17.0984) (-25.6408, 16.4177) knots 0 0 0 1 2 2 2
  spline S107 degree 2 poles (-25.6408, 16.4177) (-24.1335, 15.0465) (-22.3248, 14.0449) (-21.3621, 14.0449) knots 0 0 0 1 2 2 2
  spline S108 degree 2 poles (-21.3621, 14.0449) (-20.8564, 14.0449) (-20.0979, 14.3561) (-19.8548, 14.6381) knots 0 0 0 1 2 2 2
  spline S109 degree 2 poles (-19.8548, 14.6381) (-19.6117, 14.9201) (-19.3685, 15.6592) (-19.3685, 16.1065) knots 0 0 0 1 2 2 2
  spline S110 degree 2 poles (-19.3685, 16.1065) (-19.3685, 16.5344) (-19.5825, 17.4096) (-19.7478, 17.8083) knots 0 0 0 1 2 2 2
  spline S111 degree 2 poles (-19.7478, 17.8083) (-19.8839, 18.1487) (-20.2729, 18.7807) (-20.4091, 18.9752) knots 0 0 0 1 2 2 2
  line L63 (-20.4091, 18.9752) -> (-20.4091, 19.0628)
  line L64 (-20.4091, 19.0628) -> (-18.6976, 19.0628)
  spline S112 degree 2 poles (-18.6976, 19.0628) (-18.4544, 18.5668) (-17.9779, 16.7872) (-17.9779, 15.9898) knots 0 0 0 1 2 2 2
  spline S113 degree 2 poles (-17.9779, 15.9898) (-17.9779, 14.3075) (-19.7575, 12.4112) (-21.2745, 12.4112) knots 0 0 0 1 2 2 2
  spline S114 degree 2 poles (-21.2745, 12.4112) (-21.9844, 12.4112) (-23.1708, 12.7418) (-23.6765, 13.0336) knots 0 0 0 1 2 2 2
  spline S115 degree 2 poles (-23.6765, 13.0336) (-24.2016, 13.3253) (-25.2324, 14.1713) (-25.7284, 14.6381) knots 0 0 0 1 2 2 2
  spline S116 degree 2 poles (-25.7284, 14.6381) (-26.5549, 15.3966) (-28.3248, 17.254) (-28.8402, 17.8083) knots 0 0 0 1 2 2 2
  line L65 (-28.8402, 17.8083) -> (-28.8402, 11.9153)
  line L66 (-28.8402, 11.9153) -> (-30.2308, 11.9153)
  point P0 (-50, 70)
  point P1 (-24.0898, 67.1989)
  constraints: 1 other
emboss "Emboss1" sketch "Sketch20" operation cut depth 1 direction (-1, 0, 0)
equation "\"d4\" = 0.5 * d3"
equation "\"d6\" = 0.5 * d5"
equation "\"d14\" = d13"
equation "\"d19\" = 0.5 * d18"
equation "\"d29\" = 0.5 * d28"
body "Solid1"
